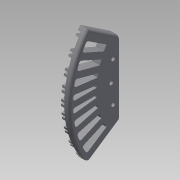
# Autodesk Inventor part: 106_CellScopeDomeBoardHolder_v4
Saved by Autodesk Inventor 2015 (Build 190159000, 159)
## iProperties
Created: 2014-07-15
Part Number: 106_CellScopeDomeBoardHolder_v4
Material: Generic
Document SubType Name: Modeling
Designer: Zack
Density: 1 g/cm^3
Appearance: Default
Author: Zack
Autodesk Inventor part; units mm, degrees
ref_plane "Work Plane1" through (50, 0, 0) normal (1, 0, 0) x (0, 1, 0)
sketch "Sketch2" plane through (50, 0, 0) normal (1, 0, 0) x (0, 1, 0)
  line L0 (-71.4127, 0) -> (71.4127, 0) projected
  line L1 (0, -15.6) -> (0, 93.6) projected
  circle A0 centre (-16, 42.5) radius 1.524
  circle A1 centre (0, 44) radius 1.524
  circle A2 centre (16, 42.5) radius 1.524
  line L2 (30, 38) -> (51.0091, 59.0091)
  arc A3 (51.0091, 59.0091) -> (-51.0091, 59.0091) centre (0, 0) ccw
  line L3 (-30, 38) -> (30, 38)
  line L4 (-30, 38) -> (-51.0091, 59.0091)
  dimension "d1" = 3.048
  dimension "d2" = 32
  dimension "d3" = 85
  dimension "d4" = 32
  dimension "d5" = 78
  dimension "d6" = 76
  dimension "d7" = 60
  dimension "d8" = 45
  dimension "d95" = 44
  constraints: 6 end point, 4 centre point, 4 point on circle, 3 point on line, 2 equal radius, 2 symmetric about line, 1 coincident, 1 horizontal
  measures "d1" diameter of A0
  measures "d2" diameter of A0.centre L1
  measures "d3" diameter of A0.centre L0
  measures "d4" diameter of A2.centre L1
  measures "d5" radius of A3
  measures "d6" diameter of L3 L0
  measures "d7" diameter of L2.start L1
  measures "d8" angle of L1 L2
  measures "d95" distance of point (0, 0) A1.centre
extrude "Extrusion1" add sketch "Sketch2" along normal blind 4.1 contours L3 L4 A3 L1 A1 | L1 A1 A3 L2 L3
sketch "Sketch3" plane through (50, 0, 0) normal (-1, 0, 0) x (0, 0, 1)
  line L0 (3.0872, -2.5) -> (0, 0)
  line L1 (0, 0) -> (71.4892, 0)
  line L2 (3.0872, 2.5) -> (0, 0)
  line L3 (72.695, -0.85) -> (65.0945, -0.85)
  line L4 (72.695, 0.85) -> (65.0945, 0.85)
  line L5 (62.6942, -0.85) -> (57.4442, -0.85)
  line L6 (57.4442, -0.85) -> (57.4442, 0.85)
  line L7 (57.4442, 0.85) -> (62.6942, 0.85)
  line L8 (77.9954, -0.85) -> (75.0952, -0.85)
  line L9 (77.9954, 0.85) -> (75.0952, 0.85)
  line L10 (77.9599, 2.5) -> (55.9442, 2.5)
  line L11 (55.9442, 2.5) -> (55.9442, -2.5)
  line L12 (55.9442, -2.5) -> (77.9599, -2.5)
  arc A0 (75.0952, -0.85) -> (75.0952, 0.85) centre (0, 0) ccw
  arc A1 (72.695, -0.85) -> (72.695, 0.85) centre (0, 0) ccw
  arc A2 (62.6942, -0.85) -> (62.6942, 0.85) centre (0, 0) ccw
  arc A3 (65.0945, -0.85) -> (65.0945, 0.85) centre (0, 0) ccw
  arc A4 (77.9599, -2.5) -> (77.9954, -0.85) centre (0, 0) ccw
  arc A5 (77.9954, 0.85) -> (77.9599, 2.5) centre (0, 0) ccw
  line L13 (72.0496, -9.703) -> (64.5057, -8.7767)
  line L14 (72.2568, -8.0156) -> (64.7128, -7.0894)
  line L15 (62.1233, -8.4842) -> (56.9125, -7.8444)
  line L16 (56.9125, -7.8444) -> (57.1196, -6.157)
  line L17 (57.1196, -6.157) -> (62.3305, -6.7968)
  line L18 (77.3104, -10.3489) -> (74.4319, -9.9955)
  line L19 (77.5176, -8.6616) -> (74.639, -8.3081)
  line L20 (77.6835, -7.0196) -> (55.8319, -4.3365)
  line L21 (55.8319, -4.3365) -> (55.2226, -9.2993)
  line L22 (55.2226, -9.2993) -> (77.0742, -11.9823)
  arc A6 (74.4319, -9.9955) -> (74.639, -8.3081) centre (0, 0) ccw
  arc A7 (72.0496, -9.703) -> (72.2568, -8.0156) centre (0, 0) ccw
  arc A8 (62.1233, -8.4842) -> (62.3305, -6.7968) centre (0, 0) ccw
  arc A9 (64.5057, -8.7767) -> (64.7128, -7.0894) centre (0, 0) ccw
  arc A10 (77.0742, -11.9823) -> (77.3104, -10.3489) centre (0, 0) ccw
  arc A11 (77.5176, -8.6616) -> (77.6835, -7.0196) centre (0, 0) ccw
  line L23 (55.2226, 9.2993) -> (77.0742, 11.9823)
  line L24 (77.6835, 7.0196) -> (55.8319, 4.3365)
  arc A12 (74.639, 8.3081) -> (74.4319, 9.9955) centre (0, 0) ccw
  line L25 (77.3104, 10.3489) -> (74.4319, 9.9955)
  arc A13 (77.3104, 10.3489) -> (77.0742, 11.9823) centre (0, 0) ccw
  arc A14 (77.6835, 7.0196) -> (77.5176, 8.6616) centre (0, 0) ccw
  line L26 (77.5176, 8.6616) -> (74.639, 8.3081)
  line L27 (56.9125, 7.8444) -> (57.1196, 6.157)
  line L28 (57.1196, 6.157) -> (62.3305, 6.7968)
  line L29 (62.1233, 8.4842) -> (56.9125, 7.8444)
  line L30 (72.0496, 9.703) -> (64.5057, 8.7767)
  line L31 (72.2568, 8.0156) -> (64.7128, 7.0894)
  arc A15 (62.3305, 6.7968) -> (62.1233, 8.4842) centre (0, 0) ccw
  arc A16 (64.7128, 7.0894) -> (64.5057, 8.7767) centre (0, 0) ccw
  arc A17 (72.2568, 8.0156) -> (72.0496, 9.703) centre (0, 0) ccw
  line L32 (55.8319, 4.3365) -> (55.2226, 9.2993)
  arc A18 (47.5, -15.6125) -> (50, 0) centre (0, 0) ccw
  line L33 (47.5, -28) -> (47.5, -15.6125)
  arc A19 (45.5, -30) -> (47.5, -28) centre (45.5, -28) ccw
  line L34 (38, -30) -> (45.5, -30)
  line L35 (49.5272, 16) -> (49.5272, 15.8447)
  arc A20 (51.4806, 16.3019) -> (49.5272, 16) centre (50.5272, 16) ccw
  line L36 (53.9421, 2.5) -> (51.9399, 2.5)
  arc A21 (53.9421, 2.5) -> (51.4806, 16.3019) centre (0, 0) ccw
  arc A22 (51.9399, 2.5) -> (49.5272, 15.8447) centre (0, 0) ccw
  line L37 (75.9506, -17.7627) -> (54.685, -12.0646)
  line L38 (55.7069, -14.0466) -> (60.778, -15.4054)
  line L39 (60.338, -17.0475) -> (55.2669, -15.6887)
  line L40 (69.998, -19.6359) -> (62.6564, -17.6687)
  line L41 (70.438, -17.9938) -> (63.0964, -16.0266)
  line L42 (53.3909, -16.8942) -> (74.6565, -22.5923)
  line L43 (75.1177, -21.0077) -> (72.3164, -20.2571)
  line L44 (75.5577, -19.3656) -> (72.7564, -18.615)
  line L45 (72.2368, -29.4253) -> (52.1244, -20.4707)
  line L46 (71.598, -30.9471) -> (68.9486, -29.7675)
  line L47 (70.9066, -32.5001) -> (68.2571, -31.3205)
  line L48 (50.0908, -25.0384) -> (70.2031, -33.993)
  line L49 (66.0645, -30.3442) -> (59.121, -27.2528)
  line L50 (66.7559, -28.7912) -> (59.8125, -25.6998)
  line L51 (52.8236, -22.5882) -> (57.6198, -24.7235)
  line L52 (56.9283, -26.2766) -> (52.1322, -24.1412)
  line L53 (48.3711, -30.9968) -> (52.749, -33.8945)
  line L54 (51.8107, -35.3121) -> (47.4328, -32.4144)
  line L55 (66.3895, -40.9443) -> (48.0309, -28.793)
  line L56 (45.2713, -32.9624) -> (63.6298, -45.1137)
  line L57 (60.1502, -40.8319) -> (53.8122, -36.6368)
  line L58 (61.0885, -39.4143) -> (54.7505, -35.2192)
  line L59 (64.5701, -43.7573) -> (62.1517, -42.1566)
  line L60 (65.5084, -42.3397) -> (63.09, -40.739)
  line L61 (75.9506, 17.7627) -> (54.685, 12.0646)
  line L62 (75.5577, 19.3656) -> (72.7564, 18.615)
  line L63 (75.1177, 21.0077) -> (72.3164, 20.2571)
  line L64 (53.3909, 16.8942) -> (74.6565, 22.5923)
  line L65 (69.998, 19.6359) -> (62.6564, 17.6687)
  line L66 (70.438, 17.9938) -> (63.0964, 16.0266)
  line L67 (55.7069, 14.0466) -> (60.778, 15.4054)
  line L68 (60.338, 17.0475) -> (55.2669, 15.6887)
  line L69 (52.8236, 22.5882) -> (57.6198, 24.7235)
  line L70 (56.9283, 26.2766) -> (52.1322, 24.1412)
  line L71 (72.2368, 29.4253) -> (52.1244, 20.4707)
  line L72 (50.0908, 25.0384) -> (70.2031, 33.993)
  line L73 (66.0645, 30.3442) -> (59.121, 27.2528)
  line L74 (66.7559, 28.7912) -> (59.8125, 25.6998)
  line L75 (70.9066, 32.5001) -> (68.2571, 31.3205)
  line L76 (71.598, 30.9471) -> (68.9486, 29.7675)
  line L77 (66.3895, 40.9443) -> (48.0309, 28.793)
  line L78 (61.0885, 39.4143) -> (54.7505, 35.2192)
  line L79 (45.2713, 32.9624) -> (63.6298, 45.1137)
  line L80 (60.1502, 40.8319) -> (53.8122, 36.6368)
  line L81 (65.5084, 42.3397) -> (63.09, 40.739)
  line L82 (64.5701, 43.7573) -> (62.1517, 42.1566)
  line L83 (48.3711, 30.9968) -> (52.749, 33.8945)
  line L84 (51.8107, 35.3121) -> (47.4328, 32.4144)
  arc A23 (53.3909, -16.8942) -> (54.685, -12.0646) centre (0, 0) ccw
  arc A24 (50.0908, -25.0384) -> (52.1244, -20.4707) centre (0, 0) ccw
  arc A25 (45.2713, -32.9624) -> (48.0309, -28.793) centre (0, 0) ccw
  arc A26 (47.4328, -32.4144) -> (48.3711, -30.9968) centre (0, 0) ccw
  arc A27 (51.8107, -35.3121) -> (52.749, -33.8945) centre (0, 0) ccw
  arc A28 (62.1517, -42.1566) -> (63.09, -40.739) centre (0, 0) ccw
  arc A29 (65.5084, -42.3397) -> (66.3895, -40.9443) centre (0, 0) ccw
  arc A30 (63.6298, -45.1137) -> (64.5701, -43.7573) centre (0, 0) ccw
  arc A31 (48.0309, 28.793) -> (45.2713, 32.9624) centre (0, 0) ccw
  arc A32 (48.3711, 30.9968) -> (47.4328, 32.4144) centre (0, 0) ccw
  arc A33 (52.749, 33.8945) -> (51.8107, 35.3121) centre (0, 0) ccw
  arc A34 (63.09, 40.739) -> (62.1517, 42.1566) centre (0, 0) ccw
  arc A35 (66.3895, 40.9443) -> (65.5084, 42.3397) centre (0, 0) ccw
  arc A36 (64.5701, 43.7573) -> (63.6298, 45.1137) centre (0, 0) ccw
  arc A37 (52.1322, -24.1412) -> (52.8236, -22.5882) centre (0, 0) ccw
  arc A38 (56.9283, -26.2766) -> (57.6198, -24.7235) centre (0, 0) ccw
  arc A39 (66.0645, -30.3442) -> (66.7559, -28.7912) centre (0, 0) ccw
  arc A40 (68.2571, -31.3205) -> (68.9486, -29.7675) centre (0, 0) ccw
  arc A41 (71.598, -30.9471) -> (72.2368, -29.4253) centre (0, 0) ccw
  arc A42 (70.2031, -33.993) -> (70.9066, -32.5001) centre (0, 0) ccw
  arc A43 (55.2669, -15.6887) -> (55.7069, -14.0466) centre (0, 0) ccw
  arc A44 (60.338, -17.0475) -> (60.778, -15.4054) centre (0, 0) ccw
  arc A45 (62.6564, -17.6687) -> (63.0964, -16.0266) centre (0, 0) ccw
  arc A46 (69.998, -19.6359) -> (70.438, -17.9938) centre (0, 0) ccw
  arc A47 (72.3164, -20.2571) -> (72.7564, -18.615) centre (0, 0) ccw
  arc A48 (75.5577, -19.3656) -> (75.9506, -17.7627) centre (0, 0) ccw
  arc A49 (74.6565, -22.5923) -> (75.1177, -21.0077) centre (0, 0) ccw
  arc A50 (59.121, -27.2528) -> (59.8125, -25.6998) centre (0, 0) ccw
  arc A51 (54.685, 12.0646) -> (53.3909, 16.8942) centre (0, 0) ccw
  arc A52 (52.1244, 20.4707) -> (50.0908, 25.0384) centre (0, 0) ccw
  arc A53 (52.8236, 22.5882) -> (52.1322, 24.1412) centre (0, 0) ccw
  arc A54 (57.6198, 24.7235) -> (56.9283, 26.2766) centre (0, 0) ccw
  arc A55 (66.7559, 28.7912) -> (66.0645, 30.3442) centre (0, 0) ccw
  arc A56 (68.9486, 29.7675) -> (68.2571, 31.3205) centre (0, 0) ccw
  arc A57 (72.2368, 29.4253) -> (71.598, 30.9471) centre (0, 0) ccw
  arc A58 (70.9066, 32.5001) -> (70.2031, 33.993) centre (0, 0) ccw
  arc A59 (55.7069, 14.0466) -> (55.2669, 15.6887) centre (0, 0) ccw
  arc A60 (60.778, 15.4054) -> (60.338, 17.0475) centre (0, 0) ccw
  arc A61 (63.0964, 16.0266) -> (62.6564, 17.6687) centre (0, 0) ccw
  arc A62 (70.438, 17.9938) -> (69.998, 19.6359) centre (0, 0) ccw
  arc A63 (72.7564, 18.615) -> (72.3164, 20.2571) centre (0, 0) ccw
  arc A64 (75.9506, 17.7627) -> (75.5577, 19.3656) centre (0, 0) ccw
  arc A65 (75.1177, 21.0077) -> (74.6565, 22.5923) centre (0, 0) ccw
  arc A66 (59.8125, 25.6998) -> (59.121, 27.2528) centre (0, 0) ccw
  arc A67 (50.0908, 25.0384) -> (48.0309, 28.793) centre (0, 0) ccw
  arc A68 (53.3909, 16.8942) -> (52.1244, 20.4707) centre (0, 0) ccw
  arc A69 (55.2226, 9.2993) -> (54.685, 12.0646) centre (0, 0) ccw
  arc A70 (54.685, -12.0646) -> (55.2226, -9.2993) centre (0, 0) ccw
  arc A71 (52.1244, -20.4707) -> (53.3909, -16.8942) centre (0, 0) ccw
  arc A72 (48.0309, -28.793) -> (50.0908, -25.0384) centre (0, 0) ccw
  arc A73 (55.9442, 2.5) -> (55.8319, 4.3365) centre (0, 0) ccw
  arc A74 (55.8319, -4.3365) -> (55.9442, -2.5) centre (0, 0) ccw
  line L85 (38, -30) -> (62.5699, -46.5726)
  arc A75 (62.5699, -46.5726) -> (63.6298, -45.1137) centre (0, 0) ccw
  arc A76 (63.6298, 45.1137) -> (62.5699, 46.5726) centre (0, 0) ccw
  line L86 (49.5272, -16) -> (49.5272, -15.8447)
  arc A77 (49.5272, -16) -> (51.4806, -16.3019) centre (50.5272, -16) ccw
  line L87 (53.9421, -2.5) -> (51.9399, -2.5)
  arc A78 (51.4806, -16.3019) -> (53.9421, -2.5) centre (0, 0) ccw
  arc A79 (49.5272, -15.8447) -> (51.9399, -2.5) centre (0, 0) ccw
  arc A80 (53.8122, -36.6368) -> (54.7505, -35.2192) centre (0, 0) ccw
  arc A81 (61.0885, 39.4143) -> (60.1502, 40.8319) centre (0, 0) ccw
  arc A82 (54.7505, 35.2192) -> (53.8122, 36.6368) centre (0, 0) ccw
  arc A83 (60.1502, -40.8319) -> (61.0885, -39.4143) centre (0, 0) ccw
  arc A84 (50, 0) -> (47.5, 15.6125) centre (0, 0) ccw
  line L88 (47.5, 28) -> (47.5, 15.6125)
  arc A85 (47.5, 28) -> (45.5, 30) centre (45.5, 28) ccw
  line L89 (38, 30) -> (45.5, 30)
  line L90 (38, 30) -> (62.5699, 46.5726)
  line L91 (38, 30) -> (38, 27.5)
  line L92 (38, -30) -> (38, 30) projected
  line L93 (38, 27.5) -> (44, 27.5)
  line L94 (46, 25.5) -> (46, 13.7113)
  arc A86 (48, 0) -> (46, 13.7113) centre (0, 0) ccw
  line L95 (38, -27.5) -> (44, -27.5)
  line L96 (46, -25.5) -> (46, -13.7113)
  arc A87 (46, -13.7113) -> (48, 0) centre (0, 0) ccw
  line L97 (38, -27.5) -> (38, -30)
  arc A88 (46, 25.5) -> (44, 27.5) centre (44, 25.5) ccw
  arc A89 (44, -27.5) -> (46, -25.5) centre (44, -25.5) ccw
  line L98 (55.3226, -9.3115) -> (55.2348, -9.1993)
  point P0 (57.4442, 94.8553)
  point P1 (3.3689, 2.1051)
  point P2 (68.576, 87.1475)
  point P3 (2.7596, -2.8576)
  point P4 (50, -25.219)
  point P5 (49.5272, 25.219)
  point P6 (50, -25.219)
  point P7 (3.6291, 1.6158)
  point P8 (2.335, -3.2139)
  point P9 (3.8372, 1.0282)
  point P10 (1.8035, -3.5396)
  point P11 (3.9543, 0.3808)
  point P12 (1.1946, -3.7887)
  point P13 (45.8609, 32.137)
  point P14 (46, 27.5)
  point P15 (46, -27.5)
  dimension "d17" = 39
  dimension "d18" = 39
  dimension "d25" = 1.7
  dimension "d26" = 1.7
  dimension "d28" = 5
  dimension "d31" = 78
  dimension "d32" = 78
  dimension "d39" = 7
  dimension "d87" = 1
  dimension "d96" = 7.6
  dimension "d97" = 2.4
  dimension "d98" = 2.4
  dimension "d101" = 8
  dimension "d106" = 52
  dimension "d107" = 54
  dimension "d111" = 9
  dimension "d115" = 9.5
  dimension "d117" = 75.1
  dimension "d118" = 34
  dimension "d119" = 5
  dimension "d130" = 5.25
  dimension "d131" = 1.5
  dimension "d132" = 48
  dimension "d133" = 1.5
  dimension "d134" = 2.5
  dimension "d135" = 2
  dimension "d139" = 0.1
  dimension "d140" = 0.1
  dimension "d141" = 32
  constraints: 196 end point, 181 point on circle, 90 centre point, 79 symmetric about line, 64 coincident, 25 point on line, 9 horizontal, 6 tangent, 4 perpendicular, 3 vertical, 1 collinear, 1 equal radius, 167 other
  measures "d17" angle of L1 L0
  measures "d18" angle of L2 L1
  measures "d25" distance between parallel lines of L4 L3
  measures "d26" distance between parallel lines of L7 L5
  measures "d28" distance of L10.end L11.end
  measures "d31" radius of A5
  measures "d32" radius of A4
  measures "d87" radius of A20
  measures "d96" radial gap between concentric circles of A1 A3
  measures "d97" radial gap between concentric circles of A2 A3
  measures "d98" radial gap between concentric circles of A1 A0
  measures "d106" radius of A22
  measures "d107" radius of A21
  measures "d117" radius of A0
  measures "d118" angle of L1 L85
  measures "d119" distance between parallel lines of L87 L36
  measures "d130" distance of L6.end L7.end
  measures "d131" distance between parallel lines of L11 L6
  measures "d132" radius of A86
  measures "d133" distance between parallel lines of L88 L94
  measures "d134" distance between parallel lines of L89 L93
  measures "d135" radius of A88
  measures "d139" vertical distance of A70.end L98.end
  measures "d140" horizontal distance of A70.end L98.start
  measures "d141" diameter of A20.centre L1
ref_plane "Work Plane4" through (50, -30, 38) normal (0, -1, 0) x (1, 0, 0)
extrude "Extrusion3" add sketch "Sketch3" along normal blind 2.5 contours A86 L94 A88 L93 L91 L89 A85 L88 A84 L1 | L1 A18 L33 A19 L34 L92 L95 A89 L96 A87 | A84 L88 A85 L89 L90 A76 L79 A31 A67 A52 A68 A51 A69 L32 A73 L11 L1 | L1 L11 A74 L21 A70 A23 A71 A24 A72 A25 L56 A75 L85 L34 A19 L33 A18 | L11 L10 A5 L9 A0 L8 A4 L12 | L32 L23 A13 L25 A12 L26 A14 L24 | L20 A11 L19 A6 L18 A10 L22 L98 L21 | L56 A25 L55 A29 L60 A28 L59 A30 | A36 L82 A34 L81 A35 L77 A31 L79 | A51 L64 A65 L63 A63 L62 A64 L61 | L37 A48 L44 A47 L43 A49 L42 A23 | A52 L72 A58 L75 A56 L76 A57 L71 | A24 L45 A41 L46 A40 L47 A42 L48
sketch "Sketch6" plane through (47.5, 0, 0) normal (-1, 0, 0) x (0, 0, 1)
  line L0 (0, 0) -> (110.3382, 0)
  line L1 (68.7133, 50.7164) -> (55.8138, 56.9945)
  line L2 (55.8138, 56.9945) -> (38, 30)
  line L3 (48.0309, 28.793) -> (62.6045, 38.439)
  line L4 (64.7475, 37.9097) -> (66.7615, 34.2386)
  line L5 (66.0565, 32.1468) -> (50.0908, 25.0384)
  arc A0 (50.0908, 25.0384) -> (48.0309, 28.793) centre (0, 0) ccw projected
  line L6 (70.2031, 33.993) -> (50.0908, 25.0384) projected
  line L7 (48.0309, 28.793) -> (66.3895, 40.9443) projected
  line L8 (0, 0) -> (81.8161, 44.8858)
  arc A1 (64.7475, 37.9097) -> (62.6045, 38.439) centre (63.4324, 37.1882) ccw
  arc A2 (66.0565, 32.1468) -> (66.7615, 34.2386) centre (65.4464, 33.5172) ccw
  line L9 (52.1244, 20.4707) -> (68.0825, 27.5757)
  line L10 (52.1244, 20.4707) -> (72.2368, 29.4253) projected
  arc A3 (53.3909, 16.8942) -> (52.1244, 20.4707) centre (0, 0) ccw projected
  line L11 (53.3909, 16.8942) -> (70.264, 21.4154)
  line L12 (74.6565, 22.5923) -> (53.3909, 16.8942) projected
  line L13 (71.2897, 23.365) -> (70.1065, 26.7061)
  line L14 (0, 0) -> (92.5461, 32.7723)
  arc A4 (55.2226, 9.2993) -> (54.685, 12.0646) centre (0, 0) ccw projected
  line L15 (54.685, 12.0646) -> (71.5458, 16.5824)
  line L16 (55.2226, 9.2993) -> (72.548, 11.4265)
  line L17 (54.685, 12.0646) -> (75.9506, 17.7627) projected
  line L18 (77.0742, 11.9823) -> (55.2226, 9.2993) projected
  line L19 (0, 0) -> (87.5621, 17.0204)
  line L20 (73.4065, 15.4198) -> (73.8376, 13.2016)
  arc A5 (55.9442, 2.5) -> (55.8319, 4.3365) centre (0, 0) ccw projected
  line L21 (55.8319, 4.3365) -> (73.1503, 6.463)
  line L22 (73.3927, 2.5) -> (55.9442, 2.5)
  line L23 (55.8319, 4.3365) -> (77.6835, 7.0196) projected
  line L24 (77.9599, 2.5) -> (55.9442, 2.5) projected
  line L25 (0, 0) -> (101.0992, 6.1835)
  line L26 (74.8303, 5.0657) -> (74.8899, 4.0916)
  arc A6 (70.1065, 26.7061) -> (68.0825, 27.5757) centre (68.6926, 26.2054) ccw
  arc A7 (70.264, 21.4154) -> (71.2897, 23.365) centre (69.8757, 22.8642) ccw
  arc A8 (73.4065, 15.4198) -> (71.5458, 16.5824) centre (71.934, 15.1336) ccw
  arc A9 (72.548, 11.4265) -> (73.8376, 13.2016) centre (72.3652, 12.9154) ccw
  arc A10 (74.8303, 5.0657) -> (73.1503, 6.463) centre (73.3331, 4.9741) ccw
  arc A11 (73.3927, 2.5) -> (74.8899, 4.0916) centre (73.3927, 4) ccw
  arc A12 (50.0908, 25.0384) -> (48.0309, 28.793) centre (0, 0) ccw
  arc A13 (53.3909, 16.8942) -> (52.1244, 20.4707) centre (0, 0) ccw
  arc A14 (55.2226, 9.2993) -> (54.685, 12.0646) centre (0, 0) ccw
  arc A15 (55.9442, 2.5) -> (55.8319, 4.3365) centre (0, 0) ccw
  line L27 (48.0309, -28.793) -> (62.6045, -38.439)
  line L28 (64.7475, -37.9097) -> (66.7615, -34.2386)
  line L29 (66.0565, -32.1468) -> (50.0908, -25.0384)
  arc A16 (62.6045, -38.439) -> (64.7475, -37.9097) centre (63.4324, -37.1882) ccw
  arc A17 (66.7615, -34.2386) -> (66.0565, -32.1468) centre (65.4464, -33.5172) ccw
  line L30 (52.1244, -20.4707) -> (68.0825, -27.5757)
  arc A18 (52.1244, -20.4707) -> (53.3909, -16.8942) centre (0, 0) ccw
  line L31 (53.3909, -16.8942) -> (70.264, -21.4154)
  line L32 (71.2897, -23.365) -> (70.1065, -26.7061)
  line L33 (54.685, -12.0646) -> (71.5458, -16.5824)
  line L34 (55.2226, -9.2993) -> (72.548, -11.4265)
  line L35 (73.4065, -15.4198) -> (73.8376, -13.2016)
  line L36 (55.8319, -4.3365) -> (73.1503, -6.463)
  line L37 (73.3927, -2.5) -> (55.9442, -2.5)
  line L38 (74.8303, -5.0657) -> (74.8899, -4.0916)
  arc A19 (68.0825, -27.5757) -> (70.1065, -26.7061) centre (68.6926, -26.2054) ccw
  arc A20 (71.2897, -23.365) -> (70.264, -21.4154) centre (69.8757, -22.8642) ccw
  arc A21 (71.5458, -16.5824) -> (73.4065, -15.4198) centre (71.934, -15.1336) ccw
  arc A22 (73.8376, -13.2016) -> (72.548, -11.4265) centre (72.3652, -12.9154) ccw
  arc A23 (73.1503, -6.463) -> (74.8303, -5.0657) centre (73.3331, -4.9741) ccw
  arc A24 (74.8899, -4.0916) -> (73.3927, -2.5) centre (73.3927, -4) ccw
  arc A25 (54.685, -12.0646) -> (55.2226, -9.2993) centre (0, 0) ccw
  arc A26 (55.8319, -4.3365) -> (55.9442, -2.5) centre (0, 0) ccw
  line L39 (50.0908, -25.0384) -> (48.0309, -28.793)
  line L40 (68.7133, 50.7164) -> (38, 30)
  line L41 (38, -30) -> (62.5699, -46.5726) projected
  line L42 (68.7133, -50.7164) -> (55.8138, -56.9945)
  line L43 (55.8138, -56.9945) -> (38, -30)
  line L44 (68.7133, -50.7164) -> (38, -30)
  point P0 (50.9444, -28.7633)
  point P1 (61.6135, -41.6746)
  point P2 (54.8167, -20.4397)
  point P3 (67.3742, -31.5231)
  point P4 (57.3393, -11.6128)
  point P5 (71.4761, -20.5953)
  point P6 (58.45, -2.5)
  point P7 (73.8179, -9.1604)
  point P8 (58.1215, 6.6744)
  point P9 (74.3421, 2.5)
  point P10 (56.3618, 15.6844)
  point P11 (73.0357, 14.0989)
  point P12 (53.2143, 24.3082)
  point P13 (69.931, 25.3506)
  point P14 (48.7565, 32.3335)
  point P15 (65.1043, 35.9781)
  point P16 (77.9599, -2.5)
  dimension "d70" = 63
  dimension "d120" = 75
  dimension "d121" = 1.5
  dimension "d122" = 75
  dimension "d123" = 75
  dimension "d124" = 75
  dimension "d125" = 1.5
  dimension "d137" = 37.0469
  dimension "d138" = 34
  constraints: 80 end point, 46 point on circle, 43 symmetric about line, 23 centre point, 16 tangent, 8 collinear, 6 equal radius, 4 perpendicular, 1 coincident, 1 horizontal, 62 other
  measures "d120" distance from line of L4 L8.start
  measures "d121" radius of A1
  measures "d122" distance from line of L0.start L13
  measures "d123" distance from line of L0.start L20
  measures "d124" distance from line of L0.start L26
  measures "d125" radius of A6
  measures "d137" distance of L1.start L2.end
  measures "d138" angle of L0 L40
extrude "Extrusion6" cut sketch "Sketch6" against normal through all
ref_plane "Work Plane5" through (0, -30, 0) normal (0, 1, 0) x (-1, 0, 0)
fillet "Fillet6" radius 2 1 edges at (54.1, 0, 78)
fillet "Fillet6" radius 2 4 edges at (54.1, -38.2863, 50.2849) (54.1, 38.2863, 50.2849) (48.75, -46.5726, 62.5699) (52.05, -46.5726, 62.5699)
sketch "Sketch9" plane through (50, 0, 0) normal (-1, 0, 0) x (0, 0, 1)
  line L0 (38, 27.5) -> (44, 27.5) projected
  arc A0 (46, 25.5) -> (44, 27.5) centre (44, 25.5) ccw projected
  line L1 (46, 25.5) -> (46, 13.7113) projected
  arc A1 (46, -13.7113) -> (46, 13.7113) centre (0, 0) ccw projected
  line L2 (46, -13.7113) -> (46, -25.5) projected
  arc A2 (44, -27.5) -> (46, -25.5) centre (44, -25.5) ccw projected
  line L3 (44, -27.5) -> (38, -27.5) projected
  line L4 (38, 27.5) -> (38, -27.5)
  point P0 (0, 0)
  constraints: 2 end point, 1 vertical
extrude "Extrusion8" cut sketch "Sketch9" against normal blind 0.1
body "Solid1"
